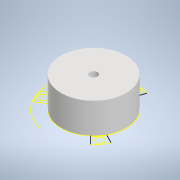
# Autodesk Inventor part: Knob
Saved by Autodesk Inventor 2022 (Build 260153000, 153)
## iProperties
Created: 2022-04-06
Part Number: Knob
Material: Generic
Document SubType Name: Modeling
Designer: awp
Density: 1 g/cm^3
Appearance: Default
Author: awp
Autodesk Inventor part; units mm, degrees
ref_plane "YZ Plane" through (0, 0, 0) normal (1, 0, 0) x (0, 1, 0)
ref_plane "XZ Plane" through (0, 0, 0) normal (0, 1, 0) x (-1, 0, 0)
ref_plane "XY Plane" through (0, 0, 0) normal (0, 0, 1) x (1, 0, 0)
sketch "Sketch1" plane through (0, 0, 0) normal (0, 1, 0) x (-1, 0, 0)
  circle A0 centre (0, 0) radius 1.5
  circle A1 centre (0, 0) radius 12.7
  dimension "d0" = 3
  dimension "d1" = 25.4
  constraints: 2 centre point, 2 coincident
  measures "d0" diameter of A0
  measures "d1" diameter of A1
extrude "Extrusion1" add sketch "Sketch1" along normal blind 3
sketch "Sketch3" plane through (0, 0, 0) normal (0, -1, 0) x (1, 0, 0)
  circle A0 centre (0, 0) radius 11.1125
  circle A1 centre (0, 0) radius 12.7 projected
  circle A2 centre (0, 0) radius 1.5 projected
  circle A3 centre (0, 0) radius 12.7 projected
  circle A4 centre (0, 0) radius 1.5 projected
  circle A5 centre (0, 0) radius 12.7
  dimension "d14" = 22.225
  constraints: 2 centre point, 2 coincident, 1 concentric
  measures "d14" diameter of A0
extrude "Extrusion3" add sketch "Sketch3" along normal blind 8.858 contours A1
sketch "Sketch4" plane through (0, 0, 0) normal (0, -1, 0) x (1, 0, 0)
  circle A0 centre (0, 0) radius 1.5 projected
  circle A1 centre (0, 0) radius 1.5 projected
  line L0 (-1.4799, -0.2447) -> (-2.9799, -0.2447)
  line L1 (-2.9799, -0.2447) -> (-1.5, -0.2447)
  line L2 (-1.5, -0.2447) -> (-1.5, 7.3753)
  line L3 (-1.5, 7.3753) -> (-2.9799, 7.3753)
  line L4 (-2.9799, 7.3753) -> (-2.9799, -0.2447)
  line L5 (-2.9799, 7.3753) -> (-4.2499, 7.3753)
  line L6 (-4.2499, 7.3753) -> (-4.2499, 3.5653)
  line L7 (-4.2499, 3.5653) -> (-2.9799, 3.5653)
  line L8 (-2.9799, 3.5653) -> (-2.9799, 7.3753)
  line L9 (-1.5, 7.3753) -> (-0.23, 7.3753)
  line L10 (-0.23, 7.3753) -> (-0.23, 3.5653)
  line L11 (-0.23, 3.5653) -> (-1.5, 3.5653)
  line L12 (-1.5, 3.5653) -> (-1.5, 7.3753)
  line L13 (-2.9799, -0.2447) -> (-1.5, -0.2447)
  line L14 (-1.5, -0.2447) -> (-1.5, -7.2297)
  line L15 (-1.5, -7.2297) -> (-2.9799, -7.2297)
  line L16 (-2.9799, -7.2297) -> (-2.9799, -0.2447)
  line L17 (-2.9799, -7.2297) -> (-4.2499, -7.2297)
  line L18 (-4.2499, -7.2297) -> (-4.2499, -3.4197)
  line L19 (-4.2499, -3.4197) -> (-2.9799, -3.4197)
  line L20 (-2.9799, -3.4197) -> (-2.9799, -7.2297)
  line L21 (-1.5, -7.2297) -> (-0.23, -7.2297)
  line L22 (-0.23, -7.2297) -> (-0.23, -3.4197)
  line L23 (-0.23, -3.4197) -> (-1.5, -3.4197)
  line L24 (-1.5, -3.4197) -> (-1.5, -7.2297)
  line L25 (-2.9799, -7.2297) -> (-4.2499, -5.9597)
  line L26 (-2.9799, -7.2297) -> (-1.1839, -7.2297) construction
  point P0 (-2.9799, 3.5653)
  point P1 (-2.9799, -3.4197)
  dimension "d17" = 1.5
  dimension "d18" = 7.62
  dimension "d19" = 1.27
  dimension "d20" = 3.81
  dimension "d21" = 1.27
  dimension "d22" = 3.81
  dimension "d37" = 6.985
  dimension "d38" = 1.27
  dimension "d39" = 3.81
  dimension "d40" = 1.27
  dimension "d41" = 135
  constraints: 54 end point, 12 parallel, 8 horizontal, 6 perpendicular, 2 point on line, 1 equal length, 2 other
  measures "d17" distance of L0.start L0.end
  measures "d18" distance of L2.end L1.end
  measures "d19" distance of L7.end L6.end
  measures "d20" distance of L6.end L5.end
  measures "d21" distance of L10.end L11.end
  measures "d22" distance of L9.end L10.end
  measures "d37" distance of L13.end L14.end
  measures "d38" distance of L18.end L19.end
  measures "d39" distance of L17.end L18.end
  measures "d40" distance of L23.end L22.end
  measures "d41" angle of L26 L25
extrude "Extrusion4" add sketch "Sketch4" along normal blind 2 contours L23 L22 L21 L14 | L16 L25 L18 L19
sketch "Sketch5" plane through (0, 3, 0) normal (0, 1, 0) x (1, 0, 0)
  circle A0 centre (0, 0) radius 12.7 projected
  circle A1 centre (0, 0) radius 1.5 projected
  circle A2 centre (0, 0) radius 12.7 projected
  line L0 (0, 12.7) -> (0, 14.605)
  line L1 (0, 14.605) -> (2.0758, 12.5292)
  line L2 (0, 14.605) -> (-2.0758, 12.5292)
  line L3 (0, 14.605) -> (2.9356, 14.605) construction
  line L4 (-4.5132, 13.8902) -> (-1.8975, 12.5574)
  line L5 (-3.9245, 12.0784) -> (-4.5132, 13.8902)
  line L6 (-4.5132, 13.8902) -> (-5.8459, 11.2745)
  line L7 (-8.5846, 11.8157) -> (-5.6851, 11.3565)
  line L8 (-7.4649, 10.2745) -> (-8.5846, 11.8157)
  line L9 (-8.5846, 11.8157) -> (-9.0438, 8.9162)
  line L10 (-11.8157, 8.5846) -> (-8.9162, 9.0438)
  line L11 (-10.2745, 7.4649) -> (-11.8157, 8.5846)
  line L12 (-11.8157, 8.5846) -> (-11.3565, 5.6851)
  line L13 (-13.8902, 4.5132) -> (-11.2745, 5.8459)
  line L14 (-12.0784, 3.9245) -> (-13.8902, 4.5132)
  line L15 (-13.8902, 4.5132) -> (-12.5574, 1.8975)
  line L16 (-14.605, 0) -> (-12.5292, 2.0758)
  line L17 (-12.7, 0) -> (-14.605, 0)
  line L18 (-14.605, 0) -> (-12.5292, -2.0758)
  line L19 (-13.8902, -4.5132) -> (-12.5574, -1.8975)
  line L20 (-12.0784, -3.9245) -> (-13.8902, -4.5132)
  line L21 (-13.8902, -4.5132) -> (-11.2745, -5.8459)
  line L22 (-11.8157, -8.5846) -> (-11.3565, -5.6851)
  line L23 (-10.2745, -7.4649) -> (-11.8157, -8.5846)
  line L24 (-11.8157, -8.5846) -> (-8.9162, -9.0438)
  line L25 (-8.5846, -11.8157) -> (-9.0438, -8.9162)
  line L26 (-7.4649, -10.2745) -> (-8.5846, -11.8157)
  line L27 (-8.5846, -11.8157) -> (-5.6851, -11.3565)
  line L28 (-4.5132, -13.8902) -> (-5.8459, -11.2745)
  line L29 (-3.9245, -12.0784) -> (-4.5132, -13.8902)
  line L30 (-4.5132, -13.8902) -> (-1.8975, -12.5574)
  line L31 (0, -14.605) -> (-2.0758, -12.5292)
  line L32 (0, -12.7) -> (0, -14.605)
  line L33 (0, -14.605) -> (2.0758, -12.5292)
  line L34 (4.5132, -13.8902) -> (1.8975, -12.5574)
  line L35 (3.9245, -12.0784) -> (4.5132, -13.8902)
  line L36 (4.5132, -13.8902) -> (5.8459, -11.2745)
  line L37 (8.5846, -11.8157) -> (5.6851, -11.3565)
  line L38 (7.4649, -10.2745) -> (8.5846, -11.8157)
  line L39 (8.5846, -11.8157) -> (9.0438, -8.9162)
  line L40 (11.8157, -8.5846) -> (8.9162, -9.0438)
  line L41 (10.2745, -7.4649) -> (11.8157, -8.5846)
  line L42 (11.8157, -8.5846) -> (11.3565, -5.6851)
  line L43 (13.8902, -4.5132) -> (11.2745, -5.8459)
  line L44 (12.0784, -3.9245) -> (13.8902, -4.5132)
  line L45 (13.8902, -4.5132) -> (12.5574, -1.8975)
  line L46 (14.605, 0) -> (12.5292, -2.0758)
  line L47 (12.7, 0) -> (14.605, 0)
  line L48 (14.605, 0) -> (12.5292, 2.0758)
  line L49 (13.8902, 4.5132) -> (12.5574, 1.8975)
  line L50 (12.0784, 3.9245) -> (13.8902, 4.5132)
  line L51 (13.8902, 4.5132) -> (11.2745, 5.8459)
  line L52 (11.8157, 8.5846) -> (11.3565, 5.6851)
  line L53 (10.2745, 7.4649) -> (11.8157, 8.5846)
  line L54 (11.8157, 8.5846) -> (8.9162, 9.0438)
  line L55 (8.5846, 11.8157) -> (9.0438, 8.9162)
  line L56 (7.4649, 10.2745) -> (8.5846, 11.8157)
  line L57 (8.5846, 11.8157) -> (5.6851, 11.3565)
  line L58 (4.5132, 13.8902) -> (5.8459, 11.2745)
  line L59 (3.9245, 12.0784) -> (4.5132, 13.8902)
  line L60 (4.5132, 13.8902) -> (1.8975, 12.5574)
  point P0 (-1.9969, 12.6081)
  point P1 (-5.7953, 11.3739)
  point P2 (-9.0264, 9.0264)
  point P3 (-11.3739, 5.7953)
  point P4 (-12.6081, 1.9969)
  point P5 (-12.6081, -1.9969)
  point P6 (-11.3739, -5.7953)
  point P7 (-9.0264, -9.0264)
  point P8 (-5.7953, -11.3739)
  point P9 (-1.9969, -12.6081)
  point P10 (1.9969, -12.6081)
  point P11 (5.7953, -11.3739)
  point P12 (9.0264, -9.0264)
  point P13 (11.3739, -5.7953)
  point P14 (12.6081, -1.9969)
  point P15 (12.6081, 1.9969)
  point P16 (11.3739, 5.7953)
  point P17 (9.0264, 9.0264)
  point P18 (5.7953, 11.3739)
  point P19 (1.9969, 12.6081)
  dimension "d28" = 1.905
  dimension "d29" = 45
  dimension "d30" = 135
  dimension "d33" = 360
  constraints: 122 end point, 2 point on circle, 1 equal length, 1 horizontal, 1 vertical, 143 other
  measures "d28" distance of L0.start L0.end
  measures "d29" angle of L0 L1
  measures "d30" angle of L2 L3
extrude "Extrusion5" [suppressed]
fillet "Fillet1" [suppressed]
body "Solid1"
